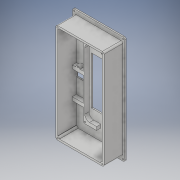
# Autodesk Inventor part: OuterDoorHousing
Saved by Autodesk Inventor 2019 (Build 230136000, 136)
## iProperties
Created: 2019-01-22
Part Number: OuterDoorHousing
Material: Generic
Document SubType Name: Modeling
Designer: garretthagen21
Density: 1 g/cm^3
Appearance: Default
Author: garretthagen21
Autodesk Inventor part; units mm, degrees
ref_plane "YZ Plane" through (0, 0, 0) normal (1, 0, 0) x (0, 1, 0)
ref_plane "XZ Plane" through (0, 0, 0) normal (0, 1, 0) x (-1, 0, 0)
ref_plane "XY Plane" through (0, 0, 0) normal (0, 0, 1) x (1, 0, 0)
sketch "Sketch1" plane through (0, 0, 0) normal (0, 0, 1) x (1, 0, 0)
  line L0 (-8.0628, -19.2011) -> (-8.0628, 77.6237)
  line L1 (-4.8878, 80.7987) -> (86.0442, 80.7987)
  line L2 (89.2192, 77.6237) -> (89.2192, -19.2011)
  line L3 (89.2192, -19.2011) -> (89.2192, -116.0259)
  line L4 (86.0442, -119.2009) -> (-4.8878, -119.2009)
  line L5 (-8.0628, -116.0259) -> (-8.0628, -19.2011)
  arc A0 (-4.8878, 80.7987) -> (-8.0628, 77.6237) centre (-4.8878, 77.6237) ccw
  arc A1 (89.2192, 77.6237) -> (86.0442, 80.7987) centre (86.0442, 77.6237) ccw
  arc A2 (-8.0628, -116.0259) -> (-4.8878, -119.2009) centre (-4.8878, -116.0259) ccw
  arc A3 (86.0442, -119.2009) -> (89.2192, -116.0259) centre (86.0442, -116.0259) ccw
  point P0 (0, 0)
  dimension "d105" = 3.175
  constraints: 12 end point, 8 point on circle, 8 tangent, 4 centre point, 3 equal radius, 3 perpendicular, 1 horizontal, 1 vertical
  measures "d105" radius of A0
extrude "Border" add sketch "Sketch1" against normal blind 2.54
sketch "Sketch5" plane through (0, 0, 0) normal (0, 0, 1) x (1, 0, 0)
  line L0 (89.2192, 102.0512) -> (89.2192, -139.2488) projected
  line L1 (-8.0628, -139.2488) -> (-8.0628, 102.0512) projected
  line L2 (77.6876, -18.5988) -> (77.6876, 25.8512)
  line L3 (77.6876, 25.8512) -> (27.294, 25.8512)
  line L4 (27.294, 25.8512) -> (27.294, -18.5988)
  line L5 (19.7883, -18.5988) -> (19.7883, -10.5978)
  line L6 (19.7883, -10.5978) -> (-0.6206, -10.5978)
  line L7 (-0.6206, -18.5988) -> (-0.6206, -26.5998)
  line L8 (-0.6206, -26.5998) -> (19.7883, -26.5998)
  line L9 (19.7883, -26.5998) -> (19.7883, -18.5988)
  line L10 (27.294, -18.5988) -> (27.294, -63.0488)
  line L11 (27.294, -63.0488) -> (77.6876, -63.0488)
  line L12 (77.6876, -63.0488) -> (77.6876, -18.5988)
  line L13 (-0.6206, -10.5978) -> (-0.6206, -18.5988)
  point P0 (0, 0)
  dimension "d33" = 44.45
  dimension "d34" = 8.001
  dimension "d35" = 8.001
  dimension "d36" = 44.45
  constraints: 24 end point, 4 perpendicular, 3 vertical, 1 parallel, 1 point on line
  measures "d33" distance of L2.start L2.end
  measures "d34" distance of L5.start L5.end
  measures "d35" distance of L7.start L7.end
  measures "d36" distance of L4.end L10.end
extrude "Screen Cutouts" cut sketch "Sketch5" against normal blind 25.4
sketch "Sketch6" plane through (0, 0, 0) normal (0, 0, 1) x (1, 0, 0)
  line L0 (27.294, 25.8512) -> (77.6876, 25.8512) projected
  line L1 (77.6876, 25.8512) -> (77.6876, -63.0488) projected
  line L2 (77.6876, -63.0488) -> (27.294, -63.0488) projected
  line L3 (27.294, -63.0488) -> (27.294, 25.8512) projected
  line L4 (-0.6206, -10.5978) -> (19.7883, -10.5978) projected
  line L5 (19.7883, -10.5978) -> (19.7883, -26.5998) projected
  line L6 (19.7883, -26.5998) -> (-0.6206, -26.5998) projected
  line L7 (-0.6206, -26.5998) -> (-0.6206, -10.5978) projected
  line L8 (81.7604, 67.1262) -> (81.7604, -104.3238)
  line L9 (-0.6206, -104.3238) -> (-0.6206, 67.1262)
  line L10 (81.777, -116.4107) -> (81.7604, -116.4107)
  line L11 (81.7604, 122.7049) -> (81.777, 122.7049)
  line L12 (2.5544, 69.5465) -> (78.5854, 69.5465)
  line L13 (2.5544, -107.9487) -> (78.5854, -107.9487)
  line L14 (-4.2528, 70.0037) -> (-4.2528, -108.4059)
  line L15 (-1.0778, -111.5809) -> (82.2342, -111.5809)
  line L16 (85.4092, -108.4059) -> (85.4092, 70.0037)
  line L17 (82.2342, 73.1787) -> (-1.0778, 73.1787)
  arc A0 (-4.2528, -108.4059) -> (-1.0778, -111.5809) centre (-1.0778, -108.4059) ccw
  arc A1 (82.2342, -111.5809) -> (85.4092, -108.4059) centre (82.2342, -108.4059) ccw
  arc A2 (-1.0778, 73.1787) -> (-4.2528, 70.0037) centre (-1.0778, 70.0037) ccw
  arc A3 (85.4092, 70.0037) -> (82.2342, 73.1787) centre (82.2342, 70.0037) ccw
  arc A4 (78.5854, -107.9487) -> (78.6435, -107.9482) centre (78.5854, -104.3238) ccw
  arc A5 (81.7209, -104.8227) -> (81.7604, -104.3238) centre (78.5854, -104.3238) ccw
  arc A6 (82.2342, -111.5809) -> (85.4092, -108.4059) centre (82.2342, -108.4059) ccw
  arc A7 (81.7209, -104.8227) -> (78.6435, -107.9482) centre (82.2342, -108.4059) ccw
  arc A8 (-4.2528, -108.4059) -> (-1.0778, -111.5809) centre (-1.0778, -108.4059) ccw
  arc A9 (2.5133, -107.9485) -> (-0.5815, -104.82) centre (-1.0778, -108.4059) ccw
  arc A10 (-0.6206, -104.3238) -> (-0.5815, -104.82) centre (2.5544, -104.3238) ccw
  arc A11 (2.5133, -107.9485) -> (2.5544, -107.9487) centre (2.5544, -104.3238) ccw
  arc A12 (-0.5815, 67.6225) -> (1.1906, 69.1257) centre (-1.0778, 70.0037) ccw
  arc A13 (-1.0778, 73.1787) -> (-4.2528, 70.0037) centre (-1.0778, 70.0037) ccw
  arc A14 (2.5544, 69.5465) -> (1.1906, 69.1257) centre (2.5544, 67.1262) ccw
  arc A15 (-0.5815, 67.6225) -> (-0.6206, 67.1262) centre (2.5544, 67.1262) ccw
  arc A16 (79.9707, 69.1108) -> (81.7209, 67.6252) centre (82.2342, 70.0037) ccw
  arc A17 (85.4092, 70.0037) -> (82.2342, 73.1787) centre (82.2342, 70.0037) ccw
  arc A18 (81.7604, 67.1262) -> (81.7209, 67.6252) centre (78.5854, 67.1262) ccw
  arc A19 (79.9707, 69.1108) -> (78.5854, 69.5465) centre (78.5854, 67.1262) ccw
  line L18 (86.0442, 80.7987) -> (-4.8878, 80.7987) projected
  line L19 (-4.8878, -119.2009) -> (86.0442, -119.2009) projected
  point P0 (0, 0)
  dimension "d39" = 3.6322
  dimension "d40" = 3.175
  dimension "d41" = 3.175
  dimension "d56" = 3.6322
  dimension "d129" = 7.62
  dimension "d130" = 7.62
  constraints: 40 point on circle, 20 centre point, 20 end point, 16 tangent, 4 coincident, 2 perpendicular, 2 point on line, 1 other
  measures "d39" distance between parallel lines of L9 L14
  measures "d40" radius of A0
  measures "d41" radius of A3
  measures "d56" distance between parallel lines of L17 L12
  measures "d129" distance between parallel lines of L18 L17
  measures "d130" distance between parallel lines of L19 L15
extrude "Outer Frame" add sketch "Sketch6" along normal blind 34.8742 contours A2 L17 A3 L16 A1 L15 A0 L14
sketch "Sketch7" plane through (0, 0, 0) normal (0, 0, 1) x (1, 0, 0)
  line L0 (77.6876, -63.0488) -> (27.294, -63.0488) projected
  line L1 (81.7604, -104.3238) -> (81.7604, 67.1262) projected
  line L2 (81.7604, -80.1938) -> (31.4684, -80.1938)
  line L3 (22.5784, -71.3038) -> (22.5784, 35.3762)
  line L4 (31.4684, 44.2662) -> (81.7604, 44.2662)
  line L5 (-0.6206, -54.8241) -> (20.0384, -54.8241)
  line L6 (20.0384, -61.1741) -> (-0.6206, -61.1741)
  line L7 (-0.6206, -26.5998) -> (-0.6206, -104.3238) projected
  line L8 (20.0384, -9.8639) -> (-0.6206, -9.8639)
  line L9 (-0.6206, -9.8639) -> (-0.6206, -22.5639)
  line L10 (-0.6206, -26.5998) -> (-0.6206, -10.5978) projected
  line L11 (-0.6206, -54.8241) -> (-0.6206, -54.8241)
  line L12 (20.0384, -80.1938) -> (20.0384, -86.5438)
  line L13 (20.0384, -86.5438) -> (81.7604, -86.5438)
  line L14 (81.7604, -86.5438) -> (81.7604, -80.1938)
  line L15 (20.0383, 37.9162) -> (20.0383, 44.2662)
  line L16 (81.7604, 44.2662) -> (81.7604, 31.5662)
  line L17 (20.0384, -61.1741) -> (20.0384, -80.1938)
  line L18 (20.0384, -9.8639) -> (20.0384, -54.8241)
  line L19 (81.7604, -86.5438) -> (81.7604, -80.1938)
  arc A0 (31.4684, 44.2662) -> (22.5784, 35.3762) centre (31.4684, 35.3762) ccw
  arc A1 (22.5784, -71.3038) -> (31.4684, -80.1938) centre (31.4684, -71.3038) ccw
  line L20 (20.0383, 44.2662) -> (20.0383, 50.6162)
  line L21 (20.0383, 50.6162) -> (81.7604, 50.6162)
  line L22 (81.7604, 44.2662) -> (81.7604, 50.6162)
  line L23 (20.0383, 37.9162) -> (20.0384, -3.4536)
  line L24 (20.0384, -9.8639) -> (20.0384, -22.5291)
  line L25 (-0.6206, -9.8639) -> (-0.6206, -3.5438)
  line L26 (81.7604, -86.5438) -> (81.7604, -80.1938)
  arc A2 (13.5189, -3.4821) -> (5.8989, -3.5153) centre (9.7089, -3.4987) ccw
  line L27 (20.0384, -3.4536) -> (13.5189, -3.4821)
  line L28 (5.8989, -3.5153) -> (-0.6206, -3.5438)
  point P0 (0, 0)
  point P1 (22.5784, -80.1938)
  point P2 (22.5784, 44.2662)
  point P3 (-0.6206, 67.1262)
  dimension "d45" = 59.182
  dimension "d46" = 124.46
  dimension "d53" = 8.89
  dimension "d61" = 6.35
  dimension "d127" = 7.62
  constraints: 50 end point, 14 point on line, 8 perpendicular, 6 collinear, 6 point on circle, 4 tangent, 4 vertical, 3 centre point, 1 equal radius, 1 horizontal
  measures "d45" distance of L2.start point (22.578, -80.194)
  measures "d46" distance of point (22.578, -80.194) point (22.578, 44.266)
  measures "d53" radius of A0
  measures "d61" distance of L15.end L20.end
  measures "d127" diameter of A2
extrude "Electronic Frame" add sketch "Sketch7" along normal blind 7.874 contours L13 L12 L17 L6 L7 L5 L18 L8 L25 L28 A2 L27 L23 L15 L20 L21 L1 L4 A0 L3 A1 L2
sketch "Sketch8" plane through (0, 0, 7.874) normal (0, 0, 1) x (1, 0, 0)
  line L0 (20.0383, 50.6162) -> (20.0383, 37.9162) projected
  line L1 (81.7604, 50.6162) -> (20.0383, 50.6162) projected
  line L2 (20.0384, -80.1938) -> (20.0384, -86.5438) projected
  line L3 (20.0384, -86.5438) -> (81.7604, -86.5438) projected
  line L4 (89.2192, -114.4511) -> (89.2192, 76.0489) projected
  line L5 (-1.7128, -120.8011) -> (82.8692, -120.8011) projected
  line L6 (-8.0628, 76.0489) -> (-8.0628, -114.4511) projected
  line L7 (82.8692, 82.3989) -> (-1.7128, 82.3989) projected
  line L8 (81.7604, 67.1262) -> (81.7604, -104.3238) projected
  line L9 (5.8989, -3.5153) -> (-0.6206, -3.5438) projected
  point P0 (0, 0)
  point P1 (23.2133, 47.4412)
  point P2 (23.2134, -83.3688)
  point P3 (78.5854, 47.4412)
  point P4 (78.5854, -83.3688)
  point P5 (9.6703, -1.9749)
  dimension "d62" = 3.175
  dimension "d63" = 3.175
  dimension "d64" = 3.175
  dimension "d65" = 3.175
  dimension "d114" = 3.175
  dimension "d115" = 3.175
  dimension "d116" = 3.175
  dimension "d117" = 3.175
  dimension "d128" = 1.524
  measures "d62" distance from line of L0 point (23.213, 47.441)
  measures "d63" distance from line of point (23.213, 47.441) L1
  measures "d64" distance from line of L2 point (23.213, -83.369)
  measures "d65" distance from line of point (23.213, -83.369) L3
  measures "d114" distance from line of L3 point (78.585, -83.369)
  measures "d115" distance from line of L8 point (78.585, -83.369)
  measures "d116" distance from line of L1 point (78.585, 47.441)
  measures "d117" distance from line of L8 point (78.585, 47.441)
  measures "d128" distance from line of L9 point (9.67, -1.975)
hole "Electronic Mounting Holes" at (23.2133, 47.4412, 7.874) at (23.2134, -83.3688, 7.874) at (78.5854, 47.4412, 7.874) at (78.5854, -83.3688, 7.874) at (9.6703, -1.9749, 7.874) direction (0, 0, -1) diameter 2.54 depth 8.89 tip angle 118
sketch "Sketch10" plane through (0, 0, 34.8742) normal (0, 0, 1) x (1, 0, 0)
  arc A0 (-1.0778, 73.1787) -> (-4.2528, 70.0037) centre (-1.0778, 70.0037) ccw projected
  arc A1 (79.9707, 69.1108) -> (81.7209, 67.6252) centre (82.2342, 70.0037) ccw projected
  arc A2 (81.7209, -104.8227) -> (78.6435, -107.9482) centre (82.2342, -108.4059) ccw projected
  arc A3 (2.5133, -107.9485) -> (-0.5815, -104.82) centre (-1.0778, -108.4059) ccw projected
  point P0 (0, 0)
  constraints: 4 coincident
hole "FrameMounting Holes" at (-1.0778, 70.0037, 34.8742) at (82.2342, 70.0037, 34.8742) at (82.2342, -108.4059, 34.8742) at (-1.0778, -108.4059, 34.8742) direction (0, 0, -1) diameter 2.54 depth 8.382 tip angle 118
sketch "Sketch11" plane through (0, 0, 7.874) normal (0, 0, 1) x (1, 0, 0)
  line L0 (31.4684, -80.1938) -> (81.7604, -80.1938) projected
  line L1 (81.7604, -80.1938) -> (81.7604, 44.2662) projected
  line L2 (81.7604, 44.2662) -> (31.4684, 44.2662) projected
  arc A0 (31.4684, 44.2662) -> (22.5784, 35.3762) centre (31.4684, 35.3762) ccw projected
  line L3 (22.5784, 35.3762) -> (22.5784, -71.3038) projected
  arc A1 (22.5784, -71.3038) -> (31.4684, -80.1938) centre (31.4684, -71.3038) ccw projected
  line L4 (27.294, 25.8512) -> (77.6876, 25.8512) projected
  line L5 (77.6876, 25.8512) -> (77.6876, -63.0488) projected
  line L6 (77.6876, -63.0488) -> (27.294, -63.0488) projected
  line L7 (27.294, -63.0488) -> (27.294, 25.8512) projected
  line L8 (31.4684, -80.1938) -> (81.7604, -80.1938) projected
  line L9 (20.0384, -86.5438) -> (81.7604, -86.5438) projected
  line L10 (52.4908, -80.1938) -> (60.4283, -80.1938)
  line L11 (60.4283, -80.1938) -> (60.4283, -86.5438)
  line L12 (60.4283, -86.5438) -> (52.4908, -86.5438)
  line L13 (52.4908, -80.1938) -> (44.5533, -80.1938)
  line L14 (44.5533, -80.1938) -> (44.5533, -86.5438)
  line L15 (44.5533, -86.5438) -> (52.4908, -86.5438)
  line L16 (31.4684, 44.2662) -> (81.7604, 44.2662) projected
  line L17 (43.6604, 44.2662) -> (43.6604, 45.5385)
  line L18 (43.6604, 45.5385) -> (30.7064, 45.5385)
  line L19 (30.7064, 45.5385) -> (30.7064, 44.2335)
  arc A2 (31.4684, 44.2662) -> (22.5784, 35.3762) centre (31.4684, 35.3762) ccw projected
  line L20 (44.5533, -86.5438) -> (60.4283, -86.5438)
  line L21 (44.5533, -80.1938) -> (60.4283, -80.1938)
  point P0 (0, 0)
  dimension "d111" = 12.954
  constraints: 22 end point, 5 perpendicular, 4 point on line, 2 collinear, 2 horizontal, 2 parallel, 1 point on circle
  measures "d111" distance of L17.end L18.end
extrude "ButtonChargerCutout" cut sketch "Sketch11" against normal blind 7.874 contours L0 L11 L9 L14 | L19 L18 L17 L2 A0
sketch "Sketch13" plane through (0, 0, 0) normal (0, 0, 1) x (1, 0, 0)
  arc A0 (-8.0628, -116.0259) -> (-4.8878, -119.2009) centre (-4.8878, -116.0259) ccw projected
  arc A1 (86.0442, -119.2009) -> (89.2192, -116.0259) centre (86.0442, -116.0259) ccw projected
  arc A2 (89.2192, 77.6237) -> (86.0442, 80.7987) centre (86.0442, 77.6237) ccw projected
  arc A3 (-4.8878, 80.7987) -> (-8.0628, 77.6237) centre (-4.8878, 77.6237) ccw projected
  point P0 (0, 0)
  constraints: 4 coincident
hole "Outer Holes" at (-4.8878, -116.0259, 0) at (86.0442, -116.0259, 0) at (86.0442, 77.6237, 0) at (-4.8878, 77.6237, 0) direction (0, 0, -1) diameter 2.54 depth 25.4 tip angle 118
fillet "Frame Fillet" radius 3.175 2 edges at (20.0384, -86.5438, 3.937) (20.0383, 50.6162, 3.937)
body "Solid1"
